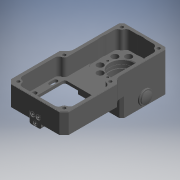
# Autodesk Inventor part: SLZ_63_Gehaeuse#
Saved by Autodesk Inventor 2017.3 (Build 213256000, 256)
## iProperties
Part Number: SLZ_63_Gehaeuse#
Material: Generic
Catalog Web Link: www.cadenas.de
Description: Antriebsgehäuse_SLZ63-Control-Tec
Vendor: ROSEKRIEGER
Document SubType Name: Modeling
Designer: partserver
Manufacturer: ROSEKRIEGER
Mass: 586.148 g
Surface Area: 1433.55 cm^2
Volume: 586.148 cm^3
Density: 1 g/cm^3
Appearance: PSOLRGB-128-128-128
Category: PARTsolutions
Company: ROSEKRIEGER
Title: SLZ_63_Gehaeuse#
Author: Cadenas PARTsolutions
Comments: Control-Tec
PSOL_IDENT_0: {$CADENAS_DATA\23d-libs\rose_krieger\linearkomponenten\pool_lineartechnik\_hubsaeule_zyliinder\elekt
PSOL_IDENT_1: rozylinder\elekzyl_slz63\parts\slz63_plfl_antrieb_gehaeuse.prj},187 {VTYP=3D},{NB=SLZ_63_Gehaeuse#},
PSOL_IDENT_2: {LINA=SLZ_63_Gehaeuse#},{NN=Antriebsgehäuse_SLZ63},{DATE=02.12.2020 11:16:23},{GEOMDATE=16.08.2018 0
PSOL_IDENT_3: 8:01:00},{VERSION=},{LINEID=10},{WBVAR=},{WBNUMERIC=}  {NB=SLZ_63_Gehaeuse#},{LINA=SLZ_63_Gehaeuse#}
PSOL_IDENT_4: ,{KT=DUMMY},{IDNR=},{CODE=TQ3},{ARTIKEL=Elektrozylinder },{TYPE=SLZ 63 KG P PL},{BEST=SLZ_63_Gehaeus
PSOL_IDENT_5: e},{VARIANTE=PL},{SPINDEL=KG 25x10},{SPINDELCODE=3.000},{SCHUTZARTVIS=IP54},{SCHUTZART=1},{HUB1=0,[0
PSOL_IDENT_6: :100]},{HINWEINBAUX=Hub + 288,5 mm},{DUMMYDURCH=10.000},{DUMMYLAENG=20.000},{HILFEHUB=105},{LAENDOPP
PSOL_IDENT_7: ROFIL=184.500},{RF=1.000},{GRUNDKOE=288.500},{A=100},{B=80},{C=100},{D=125},{E=238},{F=40},{G=M16x1.
PSOL_IDENT_8: 5},{H=104},{K=125},{L=105},{M=48},{N=56.5},{O=86},{P=18.5},{PPATH=sbl_lz70p_plfl.prj}
NB: SLZ_63_Gehaeuse#
NN: Antriebsgehäuse_SLZ63
NT: Control-Tec
NBSYN: $BEST.#
LINA: SLZ_63_Gehaeuse#
CATALOG: RK Rose+Krieger
ARTIKEL: Elektrozylinder
TYPE: SLZ 63 KG P PL
BEST: SLZ_63_Gehaeuse
VARIANTE: PL
SPINDEL: KG 25x10
SPINDELCODE: 3
SCHUTZARTVIS: IP54
SCHUTZART: 1
HUB1: 0,[0:100]
HINWEINBAUX: Hub + 288,5 mm
DUMMYDURCH: 10
DUMMYLAENG: 20
HILFEHUB: 105
LAENDOPPROFIL: 184.5
RF: 1
GRUNDKOE: 288.5
A: 100
B: 80
C: 100
D: 125
E: 238
F: 40
G: M16x1.5
H: 104
K: 125
L: 105
M: 48
N: 56.5
O: 86
P: 18.5
SUPPLIER: ROSEKRIEGER
ARTICLENO: SLZ_63_Gehaeuse#
BOMINFO: SLZ_63_Gehaeuse#
CREATOR: CADENAS GmbH
Autodesk Inventor part; units mm, degrees
sketch "Sketch_1" plane through (0, 0, 0) normal (0, 0, 1) x (1, 0, 0)
  line L0 (-61.5, -72.9142) -> (-61.5, -177.5858)
  line L1 (-61.5, -177.5858) -> (-52.0858, -187)
  line L2 (-52.0858, -187) -> (52.0858, -187)
  line L3 (52.0858, -187) -> (61.5, -177.5858)
  line L4 (61.5, -177.5858) -> (61.5, -72.9142)
  line L5 (61.5, -72.9142) -> (53.6863, -65.1005)
  arc A0 (49, -53.7868) -> (53.6863, -65.1005) centre (65, -53.7868) ccw
  line L6 (49, -53.7868) -> (49, 44.5858)
  line L7 (49, 44.5858) -> (44.5858, 49)
  line L8 (44.5858, 49) -> (-44.5858, 49)
  line L9 (-44.5858, 49) -> (-49, 44.5858)
  line L10 (-49, 44.5858) -> (-49, -53.7868)
  arc A1 (-53.6863, -65.1005) -> (-49, -53.7868) centre (-65, -53.7868) ccw
  line L11 (-53.6863, -65.1005) -> (-61.5, -72.9142)
  constraints: 24 end point, 4 point on circle, 2 centre point
extrude "Extrusion1" add sketch "Sketch_1" along normal blind 0.2
sketch "Sketch_2" plane through (0, 0, 0.2) normal (0, 0, 1) x (1, 0, 0)
  line L0 (-62.5, -178) -> (-52.5, -188)
  line L1 (-52.5, -188) -> (52.5, -188)
  line L2 (52.5, -188) -> (62.5, -178)
  line L3 (62.5, -178) -> (62.5, -72.5)
  line L4 (62.5, -72.5) -> (54.3934, -64.3934)
  arc A0 (50, -53.7868) -> (54.3934, -64.3934) centre (65, -53.7868) ccw
  line L5 (50, -53.7868) -> (50, 45)
  line L6 (50, 45) -> (45, 50)
  line L7 (45, 50) -> (-45, 50)
  line L8 (-45, 50) -> (-50, 45)
  line L9 (-50, 45) -> (-50, -53.7868)
  arc A1 (-54.3934, -64.3934) -> (-50, -53.7868) centre (-65, -53.7868) ccw
  line L10 (-54.3934, -64.3934) -> (-62.5, -72.5)
  line L11 (-62.5, -72.5) -> (-62.5, -178)
  arc A2 (43.25, -106.5) -> (51.75, -106.5) centre (47.5, -106.5) ccw
  line L12 (51.75, -106.5) -> (51.75, -96.5)
  arc A3 (51.75, -96.5) -> (43.25, -96.5) centre (47.5, -96.5) ccw
  line L13 (43.25, -96.5) -> (43.25, -106.5)
  arc A4 (43.25, -151.5) -> (51.75, -151.5) centre (47.5, -151.5) ccw
  line L14 (51.75, -151.5) -> (51.75, -141.5)
  arc A5 (51.75, -141.5) -> (43.25, -141.5) centre (47.5, -141.5) ccw
  line L15 (43.25, -141.5) -> (43.25, -151.5)
  circle A6 centre (31, 0) radius 2.45
  circle A7 centre (0, -31) radius 2.45
  arc A8 (-40, -159) -> (-35, -164) centre (-35, -159) ccw
  line L16 (-35, -164) -> (35, -164)
  arc A9 (35, -164) -> (40, -159) centre (35, -159) ccw
  line L17 (40, -159) -> (40, -89)
  arc A10 (40, -89) -> (35, -84) centre (35, -89) ccw
  line L18 (35, -84) -> (-35, -84)
  arc A11 (-35, -84) -> (-40, -89) centre (-35, -89) ccw
  line L19 (-40, -89) -> (-40, -159)
  arc A12 (-51.75, -106.5) -> (-43.25, -106.5) centre (-47.5, -106.5) ccw
  line L20 (-43.25, -106.5) -> (-43.25, -96.5)
  arc A13 (-43.25, -96.5) -> (-51.75, -96.5) centre (-47.5, -96.5) ccw
  line L21 (-51.75, -96.5) -> (-51.75, -106.5)
  arc A14 (-51.75, -151.5) -> (-43.25, -151.5) centre (-47.5, -151.5) ccw
  line L22 (-43.25, -151.5) -> (-43.25, -141.5)
  arc A15 (-43.25, -141.5) -> (-51.75, -141.5) centre (-47.5, -141.5) ccw
  line L23 (-51.75, -141.5) -> (-51.75, -151.5)
  constraints: 48 end point, 28 point on circle, 16 centre point
extrude "Extrusion2" add sketch "Sketch_2" along normal blind 83.8
sketch "Sketch_3" plane through (0, 0, 43) normal (0, 0, 1) x (1, 0, 0)
  line L0 (-72.5, -198) -> (72.5, -198)
  line L1 (72.5, -198) -> (72.5, 60)
  line L2 (72.5, 60) -> (-72.5, 60)
  line L3 (-72.5, 60) -> (-72.5, -198)
  line L4 (-50, -45) -> (-45, -50)
  line L5 (-45, -50) -> (45, -50)
  line L6 (45, -50) -> (50, -45)
  line L7 (50, -45) -> (50, 50)
  line L8 (50, 50) -> (-50, 50)
  line L9 (-50, 50) -> (-50, -45)
  constraints: 20 end point
extrude "Extrusion3" cut sketch "Sketch_3" along normal blind 41
sketch "Sketch_4" plane through (0, 0, 0) normal (0, 0, 1) x (1, 0, 0)
  line L0 (-55.5, -89.6888) -> (-55.5, -160.3112)
  arc A0 (-55.5, -160.3112) -> (-48.8423, -168.1978) centre (-47.5, -160.3112) ccw
  arc A1 (-43.1624, -174.0738) -> (-48.8423, -168.1978) centre (-50, -175) ccw
  arc A2 (-43.1624, -174.0738) -> (-35.2348, -181) centre (-35.2348, -173) ccw
  line L1 (-35.2348, -181) -> (35.2348, -181)
  arc A3 (35.2348, -181) -> (43.1624, -174.0738) centre (35.2348, -173) ccw
  arc A4 (48.8423, -168.1978) -> (43.1624, -174.0738) centre (50, -175) ccw
  arc A5 (48.8423, -168.1978) -> (55.5, -160.3112) centre (47.5, -160.3112) ccw
  line L2 (55.5, -160.3112) -> (55.5, -89.6888)
  arc A6 (55.5, -89.6888) -> (48.8423, -81.8022) centre (47.5, -89.6888) ccw
  arc A7 (43.3136, -76.7035) -> (48.8423, -81.8022) centre (50, -75) ccw
  arc A8 (43, -75) -> (43.3136, -76.7035) centre (52.9546, -74.0481) ccw
  line L3 (43, -75) -> (43, -9.3274)
  arc A9 (43, -9.3274) -> (43, 9.3274) centre (0, 0) ccw
  line L4 (43, 9.3274) -> (43, 25.964)
  arc A10 (43, 25.964) -> (37.6846, 33.5001) centre (35, 25.964) ccw
  arc A11 (33.5001, 37.6846) -> (37.6846, 33.5001) centre (40, 40) ccw
  arc A12 (33.5001, 37.6846) -> (25.964, 43) centre (25.964, 35) ccw
  line L5 (25.964, 43) -> (9.3274, 43)
  arc A13 (9.3274, 43) -> (-9.3274, 43) centre (0, 0) ccw
  line L6 (-9.3274, 43) -> (-25.964, 43)
  arc A14 (-25.964, 43) -> (-33.5001, 37.6846) centre (-25.964, 35) ccw
  arc A15 (-37.6846, 33.5001) -> (-33.5001, 37.6846) centre (-40, 40) ccw
  arc A16 (-37.6846, 33.5001) -> (-43, 25.964) centre (-35, 25.964) ccw
  line L7 (-43, 25.964) -> (-43, 9.3274)
  arc A17 (-43, 9.3274) -> (-43, -9.3274) centre (0, 0) ccw
  line L8 (-43, -9.3274) -> (-43, -75)
  arc A18 (-43.3136, -76.7035) -> (-43, -75) centre (-52.9546, -74.0481) ccw
  arc A19 (-48.8423, -81.8022) -> (-43.3136, -76.7035) centre (-50, -75) ccw
  arc A20 (-48.8423, -81.8022) -> (-55.5, -89.6888) centre (-47.5, -89.6888) ccw
  constraints: 42 point on circle, 21 centre point, 18 end point
extrude "Extrusion4" cut sketch "Sketch_4" along normal blind 37
sketch "Sketch_5" plane through (0, 0, 37) normal (0, 0, 1) x (1, 0, 0)
  arc A0 (-43, 9.3274) -> (-43, -9.3274) centre (0, 0) ccw
  line L0 (-43, -9.3274) -> (-43, -24.1039)
  arc A1 (-43, -24.1039) -> (-42.2222, -26.7822) centre (-38, -24.1039) ccw
  arc A2 (-42.2222, -26.7822) -> (42.2222, -26.7822) centre (0, 0) ccw
  arc A3 (42.2222, -26.7822) -> (43, -24.1039) centre (38, -24.1039) ccw
  line L1 (43, -24.1039) -> (43, -9.3274)
  arc A4 (43, -9.3274) -> (43, 9.3274) centre (0, 0) ccw
  line L2 (43, 9.3274) -> (43, 25.964)
  arc A5 (43, 25.964) -> (37.6846, 33.5001) centre (35, 25.964) ccw
  arc A6 (33.5001, 37.6846) -> (37.6846, 33.5001) centre (40, 40) ccw
  arc A7 (33.5001, 37.6846) -> (25.964, 43) centre (25.964, 35) ccw
  line L3 (25.964, 43) -> (9.3274, 43)
  arc A8 (9.3274, 43) -> (-9.3274, 43) centre (0, 0) ccw
  line L4 (-9.3274, 43) -> (-25.964, 43)
  arc A9 (-25.964, 43) -> (-33.5001, 37.6846) centre (-25.964, 35) ccw
  arc A10 (-37.6846, 33.5001) -> (-33.5001, 37.6846) centre (-40, 40) ccw
  arc A11 (-37.6846, 33.5001) -> (-43, 25.964) centre (-35, 25.964) ccw
  line L5 (-43, 25.964) -> (-43, 9.3274)
  constraints: 24 point on circle, 12 centre point, 12 end point
extrude "Extrusion5" cut sketch "Sketch_5" along normal blind 2
sketch "Sketch_6" plane through (0, 0, 0) normal (1, 0, 0) x (0, 0, -1)
  line L0 (-84, 0) -> (-88, 0)
  line L1 (-88, 0) -> (-88, 24.3)
  line L2 (-88, 24.3) -> (-87.5, 24.8)
  line L3 (-87.5, 24.8) -> (-84, 24.8)
  line L4 (-84, 24.8) -> (-84, 0)
  line L5 (-84, 0) -> (-88, 0)
  constraints: 12 end point
revolve "Revolution1" add sketch "Sketch_6" angle 360 about axis through (0, 0, 84) along (0, 0, -1)
sketch "Sketch_7" plane through (0, 0, 66) normal (0, 0, 1) x (1, 0, 0)
  line L0 (53, 0) -> (-53, 0)
  line L1 (-53, 0) -> (-53, 14.5)
  line L2 (-53, 14.5) -> (-52.5, 15)
  line L3 (-52.5, 15) -> (52.5, 15)
  line L4 (52.5, 15) -> (53, 14.5)
  line L5 (53, 14.5) -> (53, 0)
  line L6 (53, 0) -> (-53, 0)
  constraints: 14 end point
revolve "Revolution2" add sketch "Sketch_7" angle 360 about axis through (53, 0, 66) along (1, 0, 0)
sketch "Sketch_8" plane through (0, 0, 66) normal (0, 0, 1) x (1, 0, 0)
  line L0 (56.5008, 0) -> (53, 0)
  line L1 (53, 0) -> (53, 12)
  line L2 (53, 12) -> (54.75, 12)
  arc A0 (56.5008, 0) -> (54.75, 12) centre (14.5008, 0) ccw
  line L3 (56.5008, 0) -> (53, 0)
  constraints: 8 end point, 2 point on circle, 1 centre point
revolve "Revolution3" add sketch "Sketch_8" angle 360 about axis through (56.5008, 0, 66) along (1, 0, 0)
sketch "Sketch9" plane through (-53, 0, 66) normal (-1, 0, 0) x (0, 0, 1)
  point P0 (0, 0)
hole "Hole1" at (-53, 0, 66) direction (1, 0, 0) diameter 17.5 depth 17
sketch "Sketch_10" plane through (0, 0, 0) normal (1, 0, 0) x (0, 0, -1)
  line L0 (-39, 0) -> (-88, 0)
  line L1 (-88, 0) -> (-88, 21)
  line L2 (-88, 21) -> (-87, 20)
  line L3 (-87, 20) -> (-79, 20)
  line L4 (-79, 20) -> (-79, 25.4)
  arc A0 (-78.4, 26) -> (-79, 25.4) centre (-78.4, 25.4) ccw
  line L5 (-78.4, 26) -> (-72.75, 26)
  line L6 (-72.75, 26) -> (-72.75, 27.6)
  line L7 (-72.75, 27.6) -> (-70.25, 27.6)
  line L8 (-70.25, 27.6) -> (-70.25, 26)
  line L9 (-70.25, 26) -> (-56.75, 26)
  line L10 (-56.75, 26) -> (-56.75, 27.6)
  line L11 (-56.75, 27.6) -> (-54.25, 27.6)
  line L12 (-54.25, 27.6) -> (-54.25, 26)
  line L13 (-54.25, 26) -> (-48.8, 26)
  line L14 (-48.8, 26) -> (-48.55, 26.25)
  line L15 (-48.55, 26.25) -> (-40.5, 26.25)
  line L16 (-40.5, 26.25) -> (-39, 27.75)
  line L17 (-39, 27.75) -> (-39, 0)
  line L18 (-39, 0) -> (-88, 0)
  constraints: 38 end point, 2 point on circle, 1 centre point
revolve "Revolution4" cut sketch "Sketch_10" angle 360 about axis through (0, 0, 39) along (0, 0, -1)
sketch "Sketch11" plane through (0, 0, 39) normal (0, 0, -1) x (-1, 0, 0)
  point P0 (-16, 31)
hole "Hole2" at (16, 31, 39) direction (0, 0, 1) diameter 9.3 depth 45 counterbore diameter 14 counterbore depth 18
pattern_linear "Rectangular Pattern1" count 2 spacing 32 along (-1, 0, 0) count 2 spacing 62 along (0, -1, 0) of "Hole2"
sketch "Sketch12" plane through (0, 0, 39) normal (0, 0, -1) x (-1, 0, 0)
  point P0 (-31, 16)
hole "Hole3" at (31, 16, 39) direction (0, 0, 1) diameter 9.3 depth 45 counterbore diameter 14 counterbore depth 18
pattern_linear "Rectangular Pattern2" count 2 spacing 62 along (-1, 0, 0) count 2 spacing 32 along (0, -1, 0) of "Hole3"
sketch "Sketch_15" plane through (0, 0, 22) normal (0, 0, 1) x (1, 0, 0)
  line L0 (-22, -181) -> (22, -181)
  arc A0 (14, -173) -> (22, -181) centre (22, -173) ccw
  line L1 (14, -173) -> (14, -169)
  line L2 (14, -169) -> (-14, -169)
  line L3 (-14, -169) -> (-14, -173)
  arc A1 (-22, -181) -> (-14, -173) centre (-22, -173) ccw
  constraints: 8 end point, 4 point on circle, 2 centre point
extrude "Extrusion6" add sketch "Sketch_15" along normal blind 15
sketch "Sketch14" plane through (-52.5, -188, 0.2) normal (0, -1, 0) x (1, 0, 0)
  point P0 (58.5, 32.8)
hole "Hole4" at (6, -188, 33) direction (0, 1, 0) diameter 5 depth 19
sketch "Sketch15" plane through (-52.5, -188, 0.2) normal (0, -1, 0) x (1, 0, 0)
  point P0 (46.5, 32.8)
hole "Hole5" at (-6, -188, 33) direction (0, 1, 0) diameter 5 depth 19
sketch "Sketch_18" plane through (0, -188, 0) normal (0, 1, 0) x (1, 0, 0)
  line L0 (-12.75, -30) -> (-12.75, -43)
  line L1 (-12.75, -43) -> (12.75, -43)
  line L2 (12.75, -43) -> (12.75, -30)
  arc A0 (12.75, -30) -> (8.75, -26) centre (8.75, -30) ccw
  line L3 (8.75, -26) -> (-8.75, -26)
  arc A1 (-8.75, -26) -> (-12.75, -30) centre (-8.75, -30) ccw
  constraints: 8 end point, 4 point on circle, 2 centre point
extrude "Extrusion7" cut sketch "Sketch_18" along normal blind 10
sketch "Sketch17" plane through (0, 0, 0) normal (0, 0, -1) x (-1, 0, 0)
  point P0 (-40, 40)
hole "Hole6" at (40, 40, 0) direction (0, 0, 1) diameter 6.8 depth 22.25 tip angle 118
sketch "Sketch18" plane through (0, 0, 0) normal (0, 0, -1) x (-1, 0, 0)
  point P0 (40, 40)
hole "Hole7" at (-40, 40, 0) direction (0, 0, 1) diameter 6.8 depth 22.25 tip angle 118
sketch "Sketch19" plane through (0, 0, 0) normal (0, 0, -1) x (-1, 0, 0)
  point P0 (-50, -75)
hole "Hole8" at (50, -75, 0) direction (0, 0, 1) diameter 6.8 depth 22.25 tip angle 118
pattern_linear "Rectangular Pattern3" count 2 spacing 100 along (-1, 0, 0) count 2 spacing 100 along (0, -1, 0) of "Hole8"
sketch "Sketch_23" plane through (0, 0, 43) normal (0, 0, 1) x (1, 0, 0)
  line L0 (-59.7, -94.3399) -> (-59.7, -156.1601)
  arc A0 (-59.7, -156.1601) -> (-58.177, -159.837) centre (-54.5, -156.1601) ccw
  line L1 (-58.177, -159.837) -> (-34.337, -183.677)
  arc A1 (-34.337, -183.677) -> (-30.6601, -185.2) centre (-30.6601, -180) ccw
  line L2 (-30.6601, -185.2) -> (-20.75, -185.2)
  arc A2 (-20.75, -185.2) -> (-15.55, -180) centre (-20.75, -180) ccw
  line L3 (-15.55, -180) -> (-15.55, -178.2)
  arc A3 (-12.55, -175.2) -> (-15.55, -178.2) centre (-12.55, -178.2) ccw
  line L4 (-12.55, -175.2) -> (12.55, -175.2)
  arc A4 (15.55, -178.2) -> (12.55, -175.2) centre (12.55, -178.2) ccw
  line L5 (15.55, -178.2) -> (15.55, -180)
  arc A5 (15.55, -180) -> (20.75, -185.2) centre (20.75, -180) ccw
  line L6 (20.75, -185.2) -> (30.6601, -185.2)
  arc A6 (30.6601, -185.2) -> (34.337, -183.677) centre (30.6601, -180) ccw
  line L7 (34.337, -183.677) -> (58.177, -159.837)
  arc A7 (58.177, -159.837) -> (59.7, -156.1601) centre (54.5, -156.1601) ccw
  line L8 (59.7, -156.1601) -> (59.7, -94.3399)
  arc A8 (59.7, -94.3399) -> (58.177, -90.663) centre (54.5, -94.3399) ccw
  line L9 (58.177, -90.663) -> (37.579, -70.065)
  arc A9 (37.579, -70.065) -> (33.9021, -68.542) centre (33.9021, -73.742) ccw
  line L10 (33.9021, -68.542) -> (-33.9021, -68.542)
  arc A10 (-33.9021, -68.542) -> (-37.579, -70.065) centre (-33.9021, -73.742) ccw
  line L11 (-37.579, -70.065) -> (-58.177, -90.663)
  arc A11 (-58.177, -90.663) -> (-59.7, -94.3399) centre (-54.5, -94.3399) ccw
  line L12 (-57.5, -94.3399) -> (-57.5, -156.1601)
  arc A12 (-57.5, -156.1601) -> (-56.6213, -158.2814) centre (-54.5, -156.1601) ccw
  line L13 (-56.6213, -158.2814) -> (-32.7814, -182.1213)
  arc A13 (-32.7814, -182.1213) -> (-30.6601, -183) centre (-30.6601, -180) ccw
  line L14 (-30.6601, -183) -> (-20.75, -183)
  arc A14 (-20.75, -183) -> (-17.75, -180) centre (-20.75, -180) ccw
  line L15 (-17.75, -180) -> (-17.75, -178.2)
  arc A15 (-12.55, -173) -> (-17.75, -178.2) centre (-12.55, -178.2) ccw
  line L16 (-12.55, -173) -> (12.55, -173)
  arc A16 (17.75, -178.2) -> (12.55, -173) centre (12.55, -178.2) ccw
  line L17 (17.75, -178.2) -> (17.75, -180)
  arc A17 (17.75, -180) -> (20.75, -183) centre (20.75, -180) ccw
  line L18 (20.75, -183) -> (30.6601, -183)
  arc A18 (30.6601, -183) -> (32.7814, -182.1213) centre (30.6601, -180) ccw
  line L19 (32.7814, -182.1213) -> (56.6213, -158.2814)
  arc A19 (56.6213, -158.2814) -> (57.5, -156.1601) centre (54.5, -156.1601) ccw
  line L20 (57.5, -156.1601) -> (57.5, -94.3399)
  arc A20 (57.5, -94.3399) -> (56.6213, -92.2186) centre (54.5, -94.3399) ccw
  line L21 (56.6213, -92.2186) -> (36.0234, -71.6207)
  arc A21 (36.0234, -71.6207) -> (33.9021, -70.742) centre (33.9021, -73.742) ccw
  line L22 (33.9021, -70.742) -> (-33.9021, -70.742)
  arc A22 (-33.9021, -70.742) -> (-36.0234, -71.6207) centre (-33.9021, -73.742) ccw
  line L23 (-36.0234, -71.6207) -> (-56.6213, -92.2186)
  arc A23 (-56.6213, -92.2186) -> (-57.5, -94.3399) centre (-54.5, -94.3399) ccw
  constraints: 48 end point, 48 point on circle, 24 centre point
extrude "Extrusion8" cut sketch "Sketch_23" against normal blind 2
sketch "Sketch_25" plane through (0, 0, 74) normal (0, 0, 1) x (1, 0, 0)
  line L0 (30, 30) -> (30, 50)
  line L1 (30, 50) -> (35, 50)
  line L2 (35, 50) -> (34.188, 49.188)
  line L3 (34.188, 49.188) -> (34.188, 30.812)
  line L4 (34.188, 30.812) -> (35, 30)
  line L5 (35, 30) -> (30, 30)
  line L6 (30, 30) -> (30, 50)
  constraints: 14 end point
revolve "Revolution5" cut sketch "Sketch_25" angle 360 about axis through (30, 30, 74) along (0, -1, 0)
thread "Thread1" size "M10x1.5" class "6H" standard "ISO Metric profile" full length
sketch "Sketch_26" plane through (0, 0, 74) normal (0, 0, 1) x (1, 0, 0)
  line L0 (-30, 30) -> (-30, 50)
  line L1 (-30, 50) -> (-25, 50)
  line L2 (-25, 50) -> (-25.812, 49.188)
  line L3 (-25.812, 49.188) -> (-25.812, 30.812)
  line L4 (-25.812, 30.812) -> (-25, 30)
  line L5 (-25, 30) -> (-30, 30)
  line L6 (-30, 30) -> (-30, 50)
  constraints: 14 end point
revolve "Revolution6" cut sketch "Sketch_26" angle 360 about axis through (-30, 30, 74) along (0, -1, 0)
thread "Thread2" size "M10x1.5" class "6H" standard "ISO Metric profile" full length
sketch "Sketch_28" plane through (0, -188, 0) normal (0, 1, 0) x (1, 0, 0)
  line L0 (-12.5, -30) -> (-12.5, -49)
  arc A0 (-12.5, -49) -> (-8.5, -53) centre (-8.5, -49) ccw
  line L1 (-8.5, -53) -> (8.5, -53)
  arc A1 (8.5, -53) -> (12.5, -49) centre (8.5, -49) ccw
  line L2 (12.5, -49) -> (12.5, -30)
  arc A2 (12.5, -30) -> (8.5, -26) centre (8.5, -30) ccw
  line L3 (8.5, -26) -> (-8.5, -26)
  arc A3 (-8.5, -26) -> (-12.5, -30) centre (-8.5, -30) ccw
  circle A4 centre (6, -33) radius 3.3
  circle A5 centre (0, -47.5) radius 3.3
  circle A6 centre (-6, -33) radius 3.3
  constraints: 8 end point, 8 point on circle, 7 centre point
extrude "Extrusion9" add sketch "Sketch_28" along normal blind 10
sketch "Sketch_29" plane through (0, 0, 33) normal (0, 0, 1) x (1, 0, 0)
  line L0 (6, -188) -> (6, -182.5)
  line L1 (6, -182.5) -> (11.5, -182.5)
  line L2 (11.5, -182.5) -> (11.5, -188)
  line L3 (11.5, -188) -> (6, -188)
  line L4 (6, -188) -> (6, -182.5)
  constraints: 10 end point
revolve "Revolution7" cut sketch "Sketch_29" angle 360 about axis through (6, -188, 33) along (0, -1, 0)
sketch "Sketch_30" plane through (0, 0, 33) normal (0, 0, 1) x (1, 0, 0)
  line L0 (-6, -188) -> (-6, -182.5)
  line L1 (-6, -182.5) -> (-0.5, -182.5)
  line L2 (-0.5, -182.5) -> (-0.5, -188)
  line L3 (-0.5, -188) -> (-6, -188)
  line L4 (-6, -188) -> (-6, -182.5)
  constraints: 10 end point
revolve "Revolution8" cut sketch "Sketch_30" angle 360 about axis through (-6, -188, 33) along (0, -1, 0)
sketch "Sketch_31" plane through (0, 0, 47.5) normal (0, 0, 1) x (1, 0, 0)
  line L0 (0, -188) -> (0, -182.5)
  line L1 (0, -182.5) -> (5, -182.5)
  line L2 (5, -182.5) -> (5, -188)
  line L3 (5, -188) -> (0, -188)
  line L4 (0, -188) -> (0, -182.5)
  constraints: 10 end point
revolve "Revolution9" cut sketch "Sketch_31" angle 360 about axis through (0, -188, 47.5) along (0, -1, 0)
sketch "Sketch_32" plane through (0, 0, 33) normal (0, 0, 1) x (1, 0, 0)
  line L0 (6, -187.5) -> (6, -170.5)
  line L1 (6, -170.5) -> (8.0095, -170.5)
  line L2 (8.0095, -170.5) -> (8.5, -170.9905)
  line L3 (8.5, -170.9905) -> (8.5, -182.3)
  arc A0 (8.5, -182.3) -> (8.7, -182.5) centre (8.7, -182.3) ccw
  line L4 (8.7, -182.5) -> (10.05, -182.5)
  arc A1 (10.25, -182.7) -> (10.05, -182.5) centre (10.05, -182.7) ccw
  line L5 (10.25, -182.7) -> (10.25, -187)
  line L6 (10.25, -187) -> (9.75, -187.5)
  line L7 (9.75, -187.5) -> (6, -187.5)
  line L8 (6, -187.5) -> (6, -170.5)
  constraints: 18 end point, 4 point on circle, 2 centre point
revolve "Revolution10" add sketch "Sketch_32" angle 360 about axis through (6, -187.5, 33) along (0, -1, 0)
thread "Thread3" size "M5x0.8" class "6g" standard "ISO Metric profile" length 10.66
sketch "Sketch_33" plane through (0, 0, 33) normal (0, 0, 1) x (1, 0, 0)
  line L0 (-6, -187.5) -> (-6, -170.5)
  line L1 (-6, -170.5) -> (-3.9905, -170.5)
  line L2 (-3.9905, -170.5) -> (-3.5, -170.9905)
  line L3 (-3.5, -170.9905) -> (-3.5, -182.3)
  arc A0 (-3.5, -182.3) -> (-3.3, -182.5) centre (-3.3, -182.3) ccw
  line L4 (-3.3, -182.5) -> (-1.95, -182.5)
  arc A1 (-1.75, -182.7) -> (-1.95, -182.5) centre (-1.95, -182.7) ccw
  line L5 (-1.75, -182.7) -> (-1.75, -187)
  line L6 (-1.75, -187) -> (-2.25, -187.5)
  line L7 (-2.25, -187.5) -> (-6, -187.5)
  line L8 (-6, -187.5) -> (-6, -170.5)
  constraints: 18 end point, 4 point on circle, 2 centre point
revolve "Revolution11" add sketch "Sketch_33" angle 360 about axis through (-6, -187.5, 33) along (0, -1, 0)
thread "Thread4" size "M5x0.8" class "6g" standard "ISO Metric profile" length 10.66
sketch "Sketch_34" plane through (0, 0, 47.5) normal (0, 0, 1) x (1, 0, 0)
  line L0 (0, -187.5) -> (0, -170.5)
  line L1 (0, -170.5) -> (2.0095, -170.5)
  line L2 (2.0095, -170.5) -> (2.5, -170.9905)
  line L3 (2.5, -170.9905) -> (2.5, -182.3)
  arc A0 (2.5, -182.3) -> (2.7, -182.5) centre (2.7, -182.3) ccw
  line L4 (2.7, -182.5) -> (4.05, -182.5)
  arc A1 (4.25, -182.7) -> (4.05, -182.5) centre (4.05, -182.7) ccw
  line L5 (4.25, -182.7) -> (4.25, -187)
  line L6 (4.25, -187) -> (3.75, -187.5)
  line L7 (3.75, -187.5) -> (0, -187.5)
  line L8 (0, -187.5) -> (0, -170.5)
  constraints: 18 end point, 4 point on circle, 2 centre point
revolve "Revolution12" add sketch "Sketch_34" angle 360 about axis through (0, -187.5, 47.5) along (0, -1, 0)
thread "Thread5" size "M5x0.8" class "6g" standard "ISO Metric profile" length 10.66
sketch "Sketch_35" plane through (0, -187.5, 0) normal (0, 1, 0) x (1, 0, 0)
  line L0 (4, -34.1547) -> (6, -35.3094)
  line L1 (6, -35.3094) -> (8, -34.1547)
  line L2 (8, -34.1547) -> (8, -31.8453)
  line L3 (8, -31.8453) -> (6, -30.6906)
  line L4 (6, -30.6906) -> (4, -31.8453)
  line L5 (4, -31.8453) -> (4, -34.1547)
  constraints: 12 end point
extrude "Extrusion10" cut sketch "Sketch_35" along normal blind 2.5
sketch "Sketch_36" plane through (0, -187.5, 0) normal (0, 1, 0) x (1, 0, 0)
  line L0 (-8, -34.1547) -> (-6, -35.3094)
  line L1 (-6, -35.3094) -> (-4, -34.1547)
  line L2 (-4, -34.1547) -> (-4, -31.8453)
  line L3 (-4, -31.8453) -> (-6, -30.6906)
  line L4 (-6, -30.6906) -> (-8, -31.8453)
  line L5 (-8, -31.8453) -> (-8, -34.1547)
  constraints: 12 end point
extrude "Extrusion11" cut sketch "Sketch_36" along normal blind 2.5
sketch "Sketch_37" plane through (0, -187.5, 0) normal (0, 1, 0) x (1, 0, 0)
  line L0 (-2, -48.6547) -> (0, -49.8094)
  line L1 (0, -49.8094) -> (2, -48.6547)
  line L2 (2, -48.6547) -> (2, -46.3453)
  line L3 (2, -46.3453) -> (0, -45.1906)
  line L4 (0, -45.1906) -> (-2, -46.3453)
  line L5 (-2, -46.3453) -> (-2, -48.6547)
  constraints: 12 end point
extrude "Extrusion12" cut sketch "Sketch_37" along normal blind 2.5
sketch "Sketch_38" plane through (0, 0, 0) normal (1, 0, 0) x (0, 0, -1)
  circle A0 centre (-64, 0) radius 3.4
  constraints: 1 centre point
extrude "Extrusion13" cut sketch "Sketch_38" against normal blind 50
sketch "Sketch_39" plane through (0, 0, 66) normal (0, 0, 1) x (1, 0, 0)
  line L0 (-56.5008, 0) -> (-47, 0)
  line L1 (-50.8, 0) -> (-50.8, -7.5)
  line L2 (-50.8, -7.5) -> (-47, -7.5)
  line L3 (-47, -7.5) -> (-47, -9)
  line L4 (-47, -9) -> (-48, -10)
  line L5 (-48, -10) -> (-52.25, -10)
  arc A0 (-53, -10.75) -> (-52.25, -10) centre (-52.25, -10.75) ccw
  line L6 (-53, -10.75) -> (-53, -12)
  line L7 (-53, -12) -> (-54.75, -12)
  arc A1 (-56.5008, 0) -> (-54.75, -12) centre (-14.5008, 0) ccw
  line L8 (-56.5008, 0) -> (-50.8, 0)
  constraints: 18 end point, 4 point on circle, 2 centre point
revolve "Revolution13" add sketch "Sketch_39" angle 360 about axis through (-56.5008, 0, 66) along (-1, 0, 0)
sketch "Sketch_44" plane through (0, 0, 49) normal (0, 0, 1) x (1, 0, 0)
  line L0 (-30, 30) -> (-30, 50)
  line L1 (-30, 50) -> (-25, 50)
  line L2 (-25, 50) -> (-25.812, 49.188)
  line L3 (-25.812, 49.188) -> (-25.812, 30.812)
  line L4 (-25.812, 30.812) -> (-25, 30)
  line L5 (-25, 30) -> (-30, 30)
  line L6 (-30, 30) -> (-30, 50)
  constraints: 14 end point
revolve "Revolution14" cut sketch "Sketch_44" angle 360 about axis through (-30, 30, 49) along (0, -1, 0)
thread "Thread6" size "M10x1.5" class "6H" standard "ISO Metric profile" full length
sketch "Sketch_45" plane through (0, 0, 49) normal (0, 0, 1) x (1, 0, 0)
  line L0 (30, 30) -> (30, 50)
  line L1 (30, 50) -> (35, 50)
  line L2 (35, 50) -> (34.188, 49.188)
  line L3 (34.188, 49.188) -> (34.188, 30.812)
  line L4 (34.188, 30.812) -> (35, 30)
  line L5 (35, 30) -> (30, 30)
  line L6 (30, 30) -> (30, 50)
  constraints: 14 end point
revolve "Revolution15" cut sketch "Sketch_45" angle 360 about axis through (30, 30, 49) along (0, -1, 0)
thread "Thread7" size "M10x1.5" class "6H" standard "ISO Metric profile" full length
ref_plane "ANTRIEBDECKPLATTE_XY" through (0, 0, 0) normal (0, 0, 1) x (1, 0, 0)
ref_plane "ANTRIEBDECKPLATTE_YZ" through (0, 0, 0) normal (1, 0, 0) x (0, 1, 0)
ref_plane "ANTRIEBDECKPLATTE_ZX" through (0, 0, 0) normal (0, 1, 0) x (0, 0, 1)
ref_plane "ANTRIEBGEHAEUSE_XY" through (0, 0, 84) normal (0, 0, -1) x (1, 0, 0)
ref_plane "ANTRIEBGEHAEUSE_YZ" through (0, 0, 84) normal (1, 0, 0) x (0, -1, 0)
ref_plane "ANTRIEBGEHAEUSE_ZX" through (0, 0, 84) normal (0, -1, 0) x (0, 0, -1)
ref_plane "DPH1_XY" through (0, 50, 84) normal (1, 0, 0) x (0, 0, -1)
ref_plane "DPH1_YZ" through (0, 50, 84) normal (0, 0, -1) x (0, 1, 0)
ref_plane "DPH1_ZX" through (0, 50, 84) normal (0, 1, 0) x (1, 0, 0)
ref_plane "DPL1_XY" through (0, 50, 84) normal (1, 0, 0) x (0, 0, -1)
ref_plane "DPL1_YZ" through (0, 50, 84) normal (0, 0, -1) x (0, 1, 0)
ref_plane "DPL1_ZX" through (0, 50, 84) normal (0, 1, 0) x (1, 0, 0)
ref_plane "DPLHUB1_XY" through (0, 50, 84) normal (1, 0, 0) x (0, 0, -1)
ref_plane "DPLHUB1_YZ" through (0, 50, 84) normal (0, 0, -1) x (0, 1, 0)
ref_plane "DPLHUB1_ZX" through (0, 50, 84) normal (0, 1, 0) x (1, 0, 0)
ref_plane "DPM20_XY" through (0, 0, 66) normal (1, 0, 0) x (0, 0, -1)
ref_plane "DPM20_YZ" through (0, 0, 66) normal (0, 0, -1) x (0, 1, 0)
ref_plane "DPM20_ZX" through (0, 0, 66) normal (0, 1, 0) x (1, 0, 0)
ref_plane "DPO1_XY" through (0, 0, 66) normal (1, 0, 0) x (0, 0, -1)
ref_plane "DPO1_YZ" through (0, 0, 66) normal (0, 0, -1) x (0, 1, 0)
ref_plane "DPO1_ZX" through (0, 0, 66) normal (0, 1, 0) x (1, 0, 0)
ref_plane "RIEMENGETRIBE_XY" through (0, 0, 1) normal (0, 0, 1) x (1, 0, 0)
ref_plane "RIEMENGETRIBE_YZ" through (0, 0, 1) normal (1, 0, 0) x (0, 1, 0)
ref_plane "RIEMENGETRIBE_ZX" through (0, 0, 1) normal (0, 1, 0) x (0, 0, 1)
body "Solid1"
